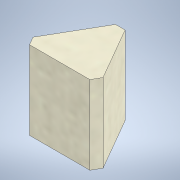
# Autodesk Inventor part: CommandToken_All
Saved by Autodesk Inventor 2021 (Build 250183000, 183)
## iProperties
Created: 2023-03-16
Part Number: CommandToken_All
Material: Paper
Document SubType Name: Modeling
Designer: Bradley
Density: 0.93 g/cm^3
Appearance: Cardboard - Chipboard
TriangleHeight: 24.800 mm
TriangleTrimmed: 21.800 mm
Author: Bradley
Autodesk Inventor part; units mm, degrees
ref_plane "YZ Plane" through (0, 0, 0) normal (1, 0, 0) x (0, 1, 0)
ref_plane "XZ Plane" through (0, 0, 0) normal (0, 1, 0) x (-1, 0, 0)
ref_plane "XY Plane" through (0, 0, 0) normal (0, 0, 1) x (1, 0, 0)
sketch "Sketch1" plane through (0, 0, 0) normal (0, 1, 0) x (-1, 0, 0)
  line L0 (1.7321, -13.5333) -> (-1.7321, -13.5333)
  line L1 (-1.7321, -13.5333) -> (-12.5862, 5.2667)
  line L2 (-12.5862, 5.2667) -> (-10.8542, 8.2667)
  line L3 (-10.8542, 8.2667) -> (10.8542, 8.2667)
  line L4 (10.8542, 8.2667) -> (12.5862, 5.2667)
  line L5 (12.5862, 5.2667) -> (1.7321, -13.5333)
  circle A0 centre (0, 0) radius 8.2667 construction
  line L6 (-1.7321, -13.5333) -> (-3.4641, -16.5333) construction
  line L7 (-3.4641, -16.5333) -> (-25.1725, -16.5333) construction
  line L8 (-25.1725, -16.5333) -> (-26.9045, -13.5333) construction
  line L9 (-26.9045, -13.5333) -> (-16.0503, 5.2667) construction
  line L10 (-16.0503, 5.2667) -> (-12.5862, 5.2667) construction
  line L11 (-28.6366, -16.5333) -> (0, -16.5333) construction
  dimension "d0" = 21.8
  dimension "d1" = 3.4641
  dimension "d4" = 24.8
  constraints: 24 end point, 9 equal length, 5 parallel, 3 horizontal, 3 tangent, 2 point on line, 1 centre point, 1 coincident, 1 collinear
  measures "d0" distance between parallel lines of L2 L5
  measures "d1" distance of L0.start L0.end
  measures "d4" distance between parallel lines of L3 L7
extrude "Extrusion1" add sketch "Sketch1" along normal mid plane 28.25
equation "\"d0\" = TriangleTrimmed"
equation "\"d4\" = TriangleHeight"
equation "\"TriangleHeight\" = 24.8"
equation "\"TriangleTrimmed\" = 21.8"
body "Solid1"
